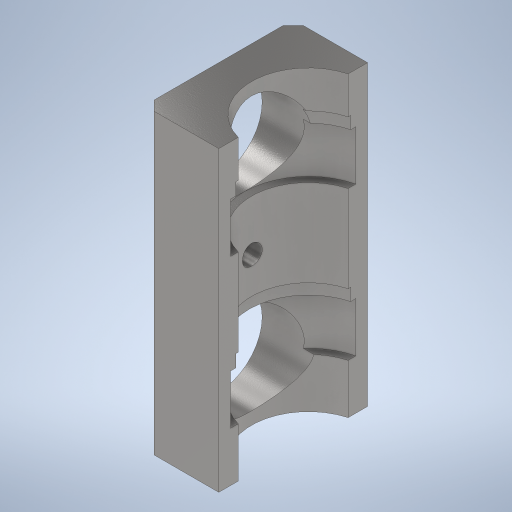
# Autodesk Inventor part: kurbelgehause
Saved by Autodesk Inventor 2024 (Build 280153000, 153)
## iProperties
Created: 2024-03-14
Part Number: kurbelgehause
Material: Stahl, galvanisiert
Document SubType Name: Modeling
Designer: ffogue
Density: 7.85 g/cm^3
Appearance: Galvanisiert
Author: ffogue
Autodesk Inventor part; units mm, degrees
note: some values were not read from the file. Chosen so that the rebuilt part matches the saved one: direction of "Bohrung1".
ref_plane "YZ Plane" through (0, 0, 0) normal (1, 0, 0) x (0, 1, 0)
sketch "Skizze1" plane through (0, 0, 0) normal (0, 0, 1) x (1, 0, 0)
  line L0 (30, 0) -> (0, 0)
  line L1 (0, 0) -> (0, 60)
  line L2 (0, 60) -> (30, 60)
  line L3 (30, 60) -> (30, 52.155)
  line L4 (30, 0) -> (30, 7.845)
  line L5 (0, 30) -> (31.8041, 30) construction
  arc A0 (30, 52.155) -> (30, 7.845) centre (36.1769, 30) ccw
  dimension "d3" = 60
  dimension "d5" = 30
  dimension "d6" = 23
  constraints: 12 end point, 2 horizontal, 2 perpendicular, 2 point on circle, 1 centre point, 1 horizontal alignment, 1 point on line, 1 symmetric about line, 1 vertical, 1 other
  measures "d3" distance between parallel lines of L0 L2
  measures "d5" distance of L1.end L2.end
  measures "d6" radius of A0
extrude "Extrusion1" add sketch "Skizze1" along normal blind 120
ref_plane "Arbeitsebene1" through (0, 0, 40) normal (0, 0, 1) x (1, 0, 0)
sketch "Skizze4" plane through (0, 0, 40) normal (0, 0, 1) x (1, 0, 0)
  circle A0 centre (36.1769, 30) radius 26
  arc A1 (30, 52.155) -> (30, 7.845) centre (36.1769, 30) ccw projected
  point P0 (0, 0)
  dimension "d20" = 52
  constraints: 1 centre point, 1 concentric
  measures "d20" diameter of A0
extrude "Extrusion5" cut sketch "Skizze4" against normal blind 20
ref_plane "Arbeitsebene2" through (0, 0, 100) normal (0, 0, 1) x (1, 0, 0)
sketch "Skizze5" plane through (0, 0, 100) normal (0, 0, 1) x (1, 0, 0)
  circle A0 centre (36.1769, 30) radius 26
  arc A1 (30, 52.155) -> (30, 7.845) centre (36.1769, 30) ccw projected
  point P0 (0, 0)
  dimension "d24" = 52
  constraints: 1 centre point, 1 concentric
  measures "d24" diameter of A0
extrude "Extrusion6" cut sketch "Skizze5" against normal blind 20
sketch "Skizze6" plane through (0, 0, 100) normal (0, 0, 1) x (1, 0, 0)
  circle A0 centre (36.1769, 30) radius 24
  arc A1 (30, 52.155) -> (30, 7.845) centre (36.1769, 30) ccw projected
  point P0 (0, 0)
  dimension "d27" = 48
  constraints: 1 centre point, 1 concentric
  measures "d27" diameter of A0
extrude "Extrusion7" cut sketch "Skizze6" along normal blind 5
sketch "Skizze7" plane through (0, 0, 40) normal (0, 0, 1) x (1, 0, 0)
  circle A0 centre (36.1769, 30) radius 24
  arc A1 (30, 52.155) -> (30, 7.845) centre (36.1769, 30) ccw projected
  point P0 (0, 0)
  dimension "d30" = 48
  constraints: 1 centre point, 1 concentric
  measures "d30" diameter of A0
extrude "Extrusion8" cut sketch "Skizze7" along normal blind 5
sketch "Skizze8" plane through (0, 0, 0) normal (-1, 0, 0) x (0, 0, 1)
  line L0 (0, 52.155) -> (0, 7.845) projected
  line L1 (0, 30) -> (120, 30) construction
  line L2 (120, 60) -> (120, 0) projected
  line L3 (0, 0) -> (120, 0) projected
  line L4 (60, 0) -> (60, 60) construction
  line L5 (0, 60) -> (120, 60) projected
  circle A0 centre (22.5, 30) radius 17.5
  circle A1 centre (97.5, 30) radius 17.5
  dimension "d33" = 75
  dimension "d34" = 35
  constraints: 4 end point, 4 midpoint, 2 centre point, 2 point on line, 1 equal radius, 1 symmetric about line
  measures "d33" distance of A1.centre A0.centre
  measures "d34" diameter of A0
extrude "Extrusion9" cut sketch "Skizze8" against normal up to surface
chamfer "Fasen1" distance 4 angle 45 2 edges at (0, 60, 60) (0, 0, 60)
sketch "Skizze10" plane through (0, 4, 0) normal (-1, 0, 0) x (0, 0, 1)
  circle A0 centre (97.5, 26) radius 17.5 projected
  circle A1 centre (22.5, 26) radius 17.5 projected
  point P0 (0, -4)
  point P1 (59.5278, 26)
  constraints: 2 horizontal alignment
hole "Bohrung1" at (0, 30, 59.5278) direction (1, 0, 0) diameter 8 end up to surface countersink diameter 12 countersink angle 90
